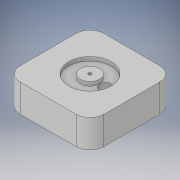
# Autodesk Inventor part: Unit_v1
Saved by Autodesk Inventor 2019 (Build 230136000, 136)
## iProperties
Created: 2018-11-20
Part Number: Unit_v1
Material: Generic
Document SubType Name: Modeling
Designer: Jeffrey Tan
Density: 1 g/cm^3
Appearance: Default
Author: Jeffrey Tan
Autodesk Inventor part; units mm, degrees
ref_plane "YZ Plane" through (0, 0, 0) normal (1, 0, 0) x (0, 1, 0)
ref_plane "XZ Plane" through (0, 0, 0) normal (0, 1, 0) x (-1, 0, 0)
ref_plane "XY Plane" through (0, 0, 0) normal (0, 0, 1) x (1, 0, 0)
sketch "Sketch1" plane through (0, 0, 0) normal (0, 1, 0) x (-1, 0, 0)
  line L0 (9.525, 9.525) -> (-9.525, 9.525)
  line L1 (-9.525, 9.525) -> (-9.525, -9.525)
  line L2 (-9.525, -9.525) -> (9.525, -9.525)
  line L3 (9.525, -9.525) -> (9.525, 9.525)
  point P0 (0, 0)
  dimension "d0" = 19.05
  dimension "d1" = 19.05
  dimension "d2" = 9.525
  dimension "d3" = 9.525
  constraints: 8 end point, 2 parallel, 1 horizontal, 1 perpendicular
  measures "d0" distance of L2.end L1.end
  measures "d1" distance of L0.end L1.end
  measures "d2" distance from line of point (0, 0) L1
  measures "d3" distance from line of L0 point (0, 0)
extrude "Extrusion1" add sketch "Sketch1" along normal blind 19.05
sketch "Sketch2" plane through (0, 0, 0) normal (0, -1, 0) x (1, 0, 0)
  line L0 (6.35, 6.35) -> (-6.35, 6.35)
  line L1 (-6.35, 6.35) -> (-6.35, -6.35)
  line L2 (-6.35, -6.35) -> (6.35, -6.35)
  line L3 (6.35, -6.35) -> (6.35, 6.35)
  point P0 (0, 0)
  dimension "d6" = 12.7
  dimension "d7" = 12.7
  dimension "d8" = 6.35
  dimension "d9" = 6.35
  constraints: 8 end point, 2 parallel, 1 horizontal, 1 perpendicular
  measures "d6" distance of L0.start L0.end
  measures "d7" distance of L2.end L0.start
  measures "d8" distance from line of point (0, 0) L3
  measures "d9" distance from line of L0 point (0, 0)
extrude "Extrusion2" cut sketch "Sketch2" against normal blind 12.7
sketch "Sketch3" plane through (0, 19.05, 0) normal (0, 1, 0) x (1, 0, 0)
  circle A0 centre (0, 0) radius 4.826
  circle A1 centre (0, 0) radius 2.159
  dimension "d12" = 9.652
  dimension "d13" = 4.318
  constraints: 2 centre point, 2 coincident
  measures "d12" diameter of A0
  measures "d13" diameter of A1
extrude "Extrusion3" cut sketch "Sketch3" against normal blind 0.889
sketch "Sketch4" plane through (0, 19.05, 0) normal (0, 1, 0) x (1, 0, 0)
  circle A0 centre (0, 0) radius 0.3619
  dimension "d16" = 0.7239
  constraints: 1 centre point, 1 coincident
  measures "d16" diameter of A0
extrude "Extrusion4" cut sketch "Sketch4" against normal through all
sketch "Sketch5" plane through (0, 18.161, 0) normal (0, 1, 0) x (1, 0, 0)
  circle A0 centre (3.4925, 0) radius 1.3335
  circle A1 centre (0, 0) radius 2.159 projected
  line L0 (0, 0) -> (3.4925, 0) construction
  dimension "d19" = 2.667
  dimension "d20" = 3.4925
  constraints: 2 end point, 1 centre point, 1 horizontal
  measures "d19" diameter of A0
  measures "d20" distance of L0.start L0.end
extrude "Extrusion5" cut sketch "Sketch5" against normal through all contours A0
sketch "Sketch7" plane through (-9.525, 0, 9.525) normal (0, 0, 1) x (1, 0, 0)
  line L0 (0, 0) -> (0, 19.05) projected
  line L1 (0, 12.7) -> (19.05, 12.7)
  line L2 (19.05, 12.7) -> (19.05, 0)
  line L3 (19.05, 0) -> (0, 0)
  line L4 (0, 0) -> (0, 12.7)
  point P0 (9.525, 0)
  dimension "d23" = 12.7
  dimension "d24" = 19.05
  constraints: 8 end point, 2 parallel, 2 point on line, 1 horizontal, 1 perpendicular
  measures "d23" distance of L1.end L2.end
  measures "d24" distance of L1.start L1.end
extrude "Extrusion6" cut sketch "Sketch7" against normal through all
fillet "Fillet1" radius 3.175 4 edges at (-9.525, 15.875, 9.525) (9.525, 15.875, 9.525) (9.525, 15.875, -9.525) (-9.525, 15.875, -9.525)
body "Solid1"
